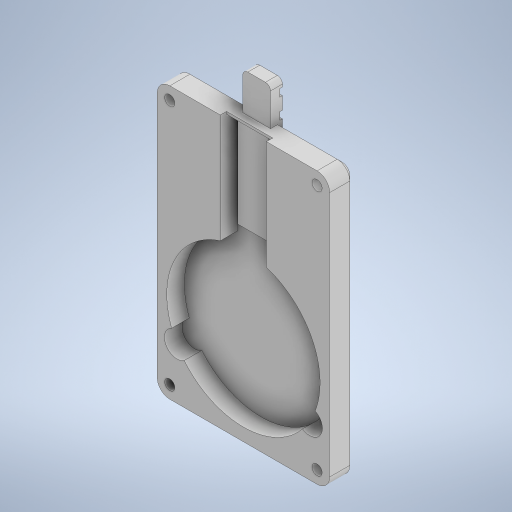
# Autodesk Inventor part: Case Back
Saved by Autodesk Inventor 2023.1 (Build 271208000, 208)
## iProperties
Created: 2022-10-09
Part Number: Case Back
Material: Generic
Document SubType Name: Modeling
Designer: Nick
Density: 1 g/cm^3
Appearance: Default
Author: Nick
Autodesk Inventor part; units mm, degrees
ref_plane "YZ Plane" through (0, 0, 0) normal (1, 0, 0) x (0, 1, 0)
ref_plane "XZ Plane" through (0, 0, 0) normal (0, 1, 0) x (-1, 0, 0)
ref_plane "XY Plane" through (0, 0, 0) normal (0, 0, 1) x (1, 0, 0)
sketch "Sketch1" plane through (0, 0, 0) normal (0, 0, 1) x (1, 0, 0)
  line L0 (0, 0) -> (68.58, 0)
  line L1 (68.58, 0) -> (68.58, 107.95)
  line L2 (68.58, 107.95) -> (0, 107.95)
  line L3 (0, 107.95) -> (0, 0)
  dimension "d0" = 68.58
  dimension "d1" = 107.95
  constraints: 8 end point, 2 parallel, 1 horizontal, 1 perpendicular
  measures "d0" distance of L2.end L1.end
  measures "d1" distance of L1.end L0.end
extrude "Extrusion1" add sketch "Sketch1" along normal blind 10
sketch "Sketch2" plane through (0, 0, 10) normal (0, 0, 1) x (1, 0, 0)
  circle A0 centre (34.29, 35.56) radius 30.48
  line L0 (0, 0) -> (68.58, 0) projected
  line L1 (68.58, 107.95) -> (0, 107.95) projected
  line L2 (25.1206, 107.95) -> (43.4594, 107.95)
  line L3 (43.4594, 107.95) -> (43.4594, 64.6281)
  line L4 (43.4594, 64.6281) -> (25.1206, 64.6281)
  line L5 (25.1206, 64.6281) -> (25.1206, 107.95)
  circle A1 centre (60.6865, 20.32) radius 5
  circle A2 centre (7.8935, 20.32) radius 5
  line L6 (7.8935, 20.32) -> (34.29, 66.04) construction
  line L7 (34.29, 66.04) -> (60.6865, 20.32) construction
  line L8 (60.6865, 20.32) -> (7.8935, 20.32) construction
  point P0 (34.29, 0)
  point P1 (34.29, 107.95)
  point P2 (57.8397, 16.2095)
  point P3 (62.8229, 24.8406)
  point P4 (10.7403, 16.2095)
  point P5 (5.7571, 24.8406)
  dimension "d4" = 18.3388
  dimension "d5" = 60.96
  dimension "d6" = 35.56
  dimension "d9" = 10
  constraints: 14 end point, 3 centre point, 3 coincident, 3 midpoint, 2 horizontal, 2 parallel, 2 point on circle, 1 equal radius, 1 perpendicular, 1 point on line, 1 vertical alignment, 7 other
  measures "d4" distance of L3.end L4.end
  measures "d5" diameter of A0
  measures "d6" distance from line of L0 A0.centre
  measures "d9" diameter of A2
extrude "Extrusion2" cut sketch "Sketch2" against normal blind 7
sketch "Sketch4" plane through (0, 0, 3) normal (0, 0, 1) x (1, 0, 0)
  arc A0 (25.1206, 64.6281) -> (5.7571, 24.8406) centre (34.29, 35.56) ccw projected
  arc A1 (5.7571, 24.8406) -> (10.7403, 16.2095) centre (7.8935, 20.32) ccw projected
  arc A2 (10.7403, 16.2095) -> (57.8397, 16.2095) centre (34.29, 35.56) ccw projected
  arc A3 (57.8397, 16.2095) -> (62.8229, 24.8406) centre (60.6865, 20.32) ccw projected
  arc A4 (62.8229, 24.8406) -> (43.4594, 64.6281) centre (34.29, 35.56) ccw projected
  line L0 (43.4594, 107.95) -> (43.4594, 64.6281) projected
  line L1 (25.1206, 107.95) -> (43.4594, 107.95) projected
  line L2 (25.1206, 64.6281) -> (25.1206, 107.95) projected
  line L3 (25.1206, 64.6281) -> (25.1206, 107.95) projected
  line L4 (43.4594, 107.95) -> (43.4594, 64.6281) projected
  line L5 (25.1206, 107.95) -> (43.4594, 107.95)
  line L6 (43.4594, 107.95) -> (43.4594, 69.85)
  line L7 (43.4594, 69.85) -> (25.1206, 69.85)
  line L8 (25.1206, 69.85) -> (25.1206, 107.95)
  line L9 (25.1206, 107.95) -> (43.4594, 107.95) projected
  line L10 (28.1206, 107.95) -> (40.4594, 107.95)
  line L11 (40.4594, 107.95) -> (40.4594, 69.85)
  line L12 (40.4594, 69.85) -> (28.1206, 69.85)
  line L13 (28.1206, 69.85) -> (28.1206, 107.95)
  point P0 (0, 0)
  dimension "d17" = 3
  dimension "d18" = 3
  dimension "d19" = 38.1
  constraints: 16 end point, 4 parallel, 2 horizontal, 2 perpendicular, 2 point on line, 1 collinear
  measures "d17" distance between parallel lines of L0 L11
  measures "d18" distance between parallel lines of L2 L13
  measures "d19" distance of L12.end L10.start
extrude "Extrusion4" add sketch "Sketch4" along normal blind 3 contours L13 L1 L11 L7
sketch "Sketch3" plane through (0, 0, 3) normal (0, 0, 1) x (1, 0, 0)
  arc A0 (25.1206, 64.6281) -> (5.7571, 24.8406) centre (34.29, 35.56) ccw projected
  arc A1 (5.7571, 24.8406) -> (10.7403, 16.2095) centre (7.8935, 20.32) ccw projected
  arc A2 (10.7403, 16.2095) -> (57.8397, 16.2095) centre (34.29, 35.56) ccw projected
  arc A3 (57.8397, 16.2095) -> (62.8229, 24.8406) centre (60.6865, 20.32) ccw projected
  arc A4 (62.8229, 24.8406) -> (43.4594, 64.6281) centre (34.29, 35.56) ccw projected
  line L0 (43.4594, 107.95) -> (43.4594, 64.6281) projected
  line L1 (25.1206, 107.95) -> (28.1206, 107.95) projected
  line L2 (25.1206, 64.6281) -> (25.1206, 107.95) projected
  line L3 (25.1206, 64.6281) -> (25.1206, 107.95) projected
  line L4 (25.1206, 107.95) -> (43.4594, 107.95)
  line L5 (43.4594, 107.95) -> (43.4594, 106.95)
  line L6 (43.4594, 106.95) -> (25.1206, 106.95)
  line L7 (25.1206, 106.95) -> (25.1206, 107.95)
  line L8 (40.4594, 107.95) -> (40.4594, 69.85) projected
  line L9 (40.4594, 69.85) -> (28.1206, 69.85) projected
  line L10 (28.1206, 69.85) -> (28.1206, 107.95) projected
  line L11 (40.4594, 107.95) -> (43.4594, 107.95) projected
  point P0 (0, 0)
  point P1 (40.4594, 106.95)
  point P2 (28.1206, 106.95)
  dimension "d10" = 1
  constraints: 8 end point, 2 parallel, 1 horizontal, 1 perpendicular, 1 point on line
  measures "d10" distance between parallel lines of L1 L6
extrude "Extrusion3" add sketch "Sketch3" along normal blind 4.5 contours L2 L1 L10 L6 | L10 L4 L8 L6 | L8 L4 L0 L6
fillet "Fillet1" radius 5 4 edges at (0, 107.95, 5) (68.58, 107.95, 5) (68.58, 0, 5) (0, 0, 5)
chamfer "Chamfer1" distance 2 angle 45 8 edges at (34.29, 107.95, 0) (1.4645, 106.4855, 0) (0, 53.975, 0) (1.4645, 1.4645, 0) (34.29, 0, 0) (67.1155, 1.4645, 0) (68.58, 53.975, 0) (67.1155, 106.4855, 0)
sketch "Sketch6" plane through (0, 0, 10) normal (0, 0, 1) x (1, 0, 0)
  arc A0 (0, 5) -> (5, 0) centre (5, 5) ccw projected
  line L0 (5, 0) -> (63.58, 0) projected
  arc A1 (63.58, 0) -> (68.58, 5) centre (63.58, 5) ccw projected
  line L1 (68.58, 5) -> (68.58, 102.95) projected
  arc A2 (68.58, 102.95) -> (63.58, 107.95) centre (63.58, 102.95) ccw projected
  line L2 (63.58, 107.95) -> (43.4594, 107.95) projected
  line L3 (43.4594, 107.95) -> (43.4594, 64.6281) projected
  arc A3 (62.8229, 24.8406) -> (43.4594, 64.6281) centre (34.29, 35.56) ccw projected
  arc A4 (57.8397, 16.2095) -> (62.8229, 24.8406) centre (60.6865, 20.32) ccw projected
  arc A5 (10.7403, 16.2095) -> (57.8397, 16.2095) centre (34.29, 35.56) ccw projected
  arc A6 (5.7571, 24.8406) -> (10.7403, 16.2095) centre (7.8935, 20.32) ccw projected
  arc A7 (25.1206, 64.6281) -> (5.7571, 24.8406) centre (34.29, 35.56) ccw projected
  line L4 (25.1206, 64.6281) -> (25.1206, 107.95) projected
  line L5 (25.1206, 107.95) -> (5, 107.95) projected
  arc A8 (5, 107.95) -> (0, 102.95) centre (5, 102.95) ccw projected
  line L6 (0, 102.95) -> (0, 5) projected
  point P0 (0, 0)
hole "Hole2" at (5, 102.95, 10) at (5, 5, 10) at (63.58, 5, 10) at (63.58, 102.95, 10) direction (0, 0, -1) diameter 4 depth 6
sketch "Sketch7" plane through (25.1206, 107.95, 7.5) normal (0, 1, 0) x (1, 0, 0)
  line L0 (3.6694, -5.25) -> (14.6694, -5.25)
  line L1 (14.6694, -5.25) -> (14.6694, 2.75)
  line L2 (14.6694, 2.75) -> (3.6694, 2.75)
  line L3 (3.6694, 2.75) -> (3.6694, -5.25)
  line L4 (-20.1206, 5.5) -> (38.4594, 5.5) projected
  line L5 (-20.1206, -2.5) -> (-20.1206, 5.5) projected
  line L6 (0, -2.5) -> (-20.1206, -2.5) projected
  line L7 (0, -2.5) -> (0, 0) projected
  line L8 (18.3388, 0) -> (0, 0) projected
  line L9 (18.3388, 0) -> (18.3388, -2.5) projected
  line L10 (38.4594, -2.5) -> (18.3388, -2.5) projected
  line L11 (38.4594, 5.5) -> (38.4594, -2.5) projected
  line L12 (38.4594, 5.5) -> (-20.1206, 5.5) projected
  line L13 (3.6694, 2.75) -> (14.6694, 2.75)
  line L14 (14.6694, 2.75) -> (14.6694, 5.5)
  line L15 (14.6694, 5.5) -> (3.6694, 5.5)
  line L16 (3.6694, 5.5) -> (3.6694, 2.75)
  line L17 (3.6694, 5.5) -> (14.6694, 5.5)
  line L18 (14.6694, 5.5) -> (14.6694, 7.5)
  line L19 (14.6694, 7.5) -> (3.6694, 7.5)
  line L20 (3.6694, 7.5) -> (3.6694, 5.5)
  line L21 (38.4594, 7.5) -> (-20.1206, 7.5) projected
  point P0 (-25.1206, 7.5)
  point P1 (3.6694, -1.25)
  point P2 (0, -1.25)
  point P3 (9.1694, 2.75)
  point P4 (9.1694, 0)
  point P5 (14.6694, 2.75)
  dimension "d36" = 8
  dimension "d37" = 11
  constraints: 24 end point, 6 parallel, 4 midpoint, 3 collinear, 3 horizontal, 3 perpendicular, 1 horizontal alignment, 1 point on line, 1 vertical alignment
  measures "d36" distance of L0.end L1.end
  measures "d37" distance of L1.end L2.end
extrude "Extrusion5" add sketch "Sketch7" along normal blind 15 and the other way blind 5 contours L16 L4 L14 L2 | L20 L19 L18 L4
sketch "Sketch8" plane through (0, 0, 0) normal (0, 0, -1) x (-1, 0, 0)
  line L0 (-28.79, 107.95) -> (-28.79, 122.95) projected
  line L1 (-39.79, 105.95) -> (-39.79, 122.95) projected
  line L2 (-28.79, 119.95) -> (-39.79, 119.95)
  line L3 (-39.79, 119.95) -> (-39.79, 116.95)
  line L4 (-39.79, 116.95) -> (-28.79, 116.95)
  line L5 (-28.79, 116.95) -> (-28.79, 119.95)
  line L6 (-28.79, 111.95) -> (-39.79, 111.95)
  line L7 (-39.79, 111.95) -> (-39.79, 108.95)
  line L8 (-39.79, 108.95) -> (-28.79, 108.95)
  line L9 (-28.79, 108.95) -> (-28.79, 111.95)
  line L10 (-5, 107.95) -> (-28.79, 107.95) projected
  line L11 (-39.79, 122.95) -> (-28.79, 122.95) projected
  point P0 (0, 0)
  dimension "d42" = 3
  dimension "d43" = 3
  dimension "d44" = 1
  dimension "d45" = 3
  constraints: 16 end point, 4 parallel, 4 point on line, 2 horizontal, 2 perpendicular
  measures "d42" distance of L3.end L2.end
  measures "d43" distance of L7.end L6.end
  measures "d44" distance between parallel lines of L8 L10
  measures "d45" distance between parallel lines of L11 L2
extrude "Extrusion6" cut sketch "Sketch8" against normal blind 1 contours L8 L1 L6 L0 | L4 L1 L2 L0
fillet "Fillet2" radius 2 2 edges at (28.79, 122.95, 2.375) (39.79, 122.95, 2.375)
body "Solid1"
